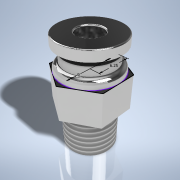
# Autodesk Inventor part: bowden-adapter-coldend
Saved by Autodesk Inventor 2021 (Build 250183000, 183)
## iProperties
Created: 2021-01-15
Part Number: bowden-adapter-coldend
Material: Aluminum 6061
Document SubType Name: Modeling
Designer: WubbGmbaa
Density: 2.7 g/cm^3
Appearance: Aluminum - Flat
Author: WubbGmbaa
Autodesk Inventor part; units mm, degrees
ref_plane "YZ Plane" through (0, 0, 0) normal (1, 0, 0) x (0, 1, 0)
ref_plane "XZ Plane" through (0, 0, 0) normal (0, 1, 0) x (-1, 0, 0)
ref_plane "XY Plane" through (0, 0, 0) normal (0, 0, 1) x (1, 0, 0)
sketch "Sketch1" plane through (0, 0, 0) normal (0, 1, 0) x (-1, 0, 0)
  line L0 (0, 0) -> (0, -6.25) construction
  line L1 (0, -6.25) -> (-5.4127, -3.125) construction
  line L2 (-5.4127, -3.125) -> (-5.4127, 3.125) construction
  line L3 (-5.4127, 3.125) -> (0, 6.25) construction
  line L4 (0, 6.25) -> (5.4127, 3.125) construction
  line L5 (5.4127, 3.125) -> (5.4127, -3.125) construction
  line L6 (5.4127, -3.125) -> (0, -6.25) construction
  line L7 (5.4127, 3.125) -> (5.4127, -3.125)
  line L8 (5.4127, -3.125) -> (0, -6.25)
  line L9 (0, -6.25) -> (-5.4127, -3.125)
  line L10 (-5.4127, -3.125) -> (-5.4127, 3.125)
  line L11 (-5.4127, 3.125) -> (0, 6.25)
  line L12 (0, 6.25) -> (5.4127, 3.125)
  circle A0 centre (0, 0) radius 4.5
  circle A1 centre (0, 0) radius 5.4127
  circle A2 centre (0, 0) radius 4
  dimension "d0" = 6.25
  dimension "d1" = 9
  dimension "d2" = 8
  constraints: 26 end point, 5 coincident, 3 centre point, 1 vertical, 26 other
  measures "d0" distance of L0.start L0.end
  measures "d1" diameter of A0
  measures "d2" diameter of A2
extrude "Extrusion1" add sketch "Sketch1" along normal blind 3 contours A0 | A2
extrude "Extrusion2" add sketch "Sketch1" along normal blind 1.5 contours A1
extrude "Extrusion3" add sketch "Sketch1" against normal blind 6 contours L7 A1 L12 | A1 | L7 L8 A1 | A1 L11 L12 | L8 L9 A1 | A1 L10 L11 | L9 L10 A1 | A0 | A2
fillet "Fillet1" radius 1 1 edges at (5.4127, 1.5, 0)
sketch "Sketch2" plane through (0, -6, 0) normal (0, -1, 0) x (1, 0, 0)
  circle A0 centre (0, 0) radius 4.5
  dimension "d10" = 9
  constraints: 1 centre point, 1 coincident
  measures "d10" diameter of A0
extrude "Extrusion4" add sketch "Sketch2" along normal blind 7.25
thread "Thread1" size "M9x1" class "6g" standard "ANSI Metric M Profile" length 7.25
sketch "Sketch3" plane through (0, 3, 0) normal (0, 1, 0) x (1, 0, 0)
  circle A0 centre (0, 0) radius 2.75
  dimension "d15" = 5.5
  constraints: 1 centre point, 1 coincident
  measures "d15" diameter of A0
extrude "Extrusion5" add sketch "Sketch3" along normal blind 1
sketch "Sketch4" plane through (0, 4, 0) normal (0, 1, 0) x (1, 0, 0)
  circle A0 centre (0, 0) radius 5.5145
  constraints: 1 centre point, 1 coincident
extrude "Extrusion6" add sketch "Sketch4" along normal blind 1.8
sketch "Sketch5" plane through (0, 5.8, 0) normal (0, 1, 0) x (1, 0, 0)
  circle A0 centre (0, 0) radius 2.25
  dimension "d20" = 4.5
  constraints: 1 centre point, 1 coincident
  measures "d20" diameter of A0
extrude "Extrusion7" cut sketch "Sketch5" against normal blind 20
fillet "Fillet2" radius 0.24 3 edges at (-5.5145, 5.8, 0) (-5.5145, 4, 0) (-2.25, 5.8, 0)
ref_plane "Work Plane1" through (0, 3, 0) normal (0, 1, 0) x (1, 0, 0)
split body "Split1" result two bodies by plane through (0, 3, 0) normal (0, 1, 0) first body at (4.2712, 5.3, 0.6194)
body "Solid2"
body "Solid3"
